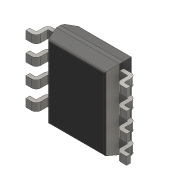
# Autodesk Inventor part: TCS3200
Saved by Autodesk Inventor 2016 (Build 200138000, 138)
## iProperties
Created: 2016-08-30
Part Number: TCS3200
Material: ABS Plastic
Document SubType Name: Modeling
Designer: Ádi
Density: 1.06 g/cm^3
Appearance: Semi-Polished
Mass: 0.0345678 g
Surface Area: 0.885583 cm^2
Volume: 0.0326111 cm^3
Author: Ádi
Autodesk Inventor part; units mm, degrees
ref_plane "YZ Plane" through (0, 0, 0) normal (1, 0, 0) x (0, 1, 0)
ref_plane "XZ Plane" through (0, 0, 0) normal (0, 1, 0) x (-1, 0, 0)
ref_plane "XY Plane" through (0, 0, 0) normal (0, 0, 1) x (1, 0, 0)
sketch "Sketch1" plane through (0, 0, 0) normal (0, 1, 0) x (-1, 0, 0)
  line L0 (-2, 2.5) -> (2, 2.5)
  line L1 (2, 2.5) -> (2, -2.5)
  line L2 (2, -2.5) -> (-2, -2.5)
  line L3 (-2, -2.5) -> (-2, 2.5)
  line L4 (-2, 2.5) -> (2, -2.5) construction
  line L5 (2, 2.5) -> (-2, -2.5) construction
  point P0 (0, 0)
  dimension "d0" = 4
  dimension "d1" = 5
  constraints: 12 end point, 2 midpoint, 2 parallel, 1 horizontal, 1 perpendicular
  measures "d0" distance of L1.end L2.end
  measures "d1" distance of L0.end L1.end
extrude "Extrusion1" add sketch "Sketch1" along normal blind 1.75
chamfer "Chamfer1" distance 0.5 angle 45 1 edges at (-2, 1.75, 0)
chamfer "Chamfer2" distance 0.2 angle 75 1 edges at (0, 0, 2.5) measured on face at (0.6667, 0, 0.8333)
chamfer "Chamfer3" distance 0.2 angle 75 1 edges at (2, 0, -0.1) measured on face at (0.6667, 0, 0.7)
chamfer "Chamfer4" distance 0.2 angle 75 1 edges at (-0.1, 0, -2.5) measured on face at (0.5333, 0, 0.7)
chamfer "Chamfer5" distance 0.2 angle 75 1 edges at (-2, 0, 0) measured on face at (0.5333, 0, 0.7667)
chamfer "Chamfer6" distance 0.2 angle 75 1 edges at (2, 1.75, 0) measured on face at (0.8333, 1.75, 0.8333)
chamfer "Chamfer7" distance 0.2 angle 75 1 edges at (0.15, 1.75, -2.5) measured on face at (0.7, 1.75, 0.8333)
chamfer "Chamfer8" distance 0.2 angle 75 1 edges at (0.15, 1.75, 2.5) measured on face at (0.7, 1.75, 0.9)
fillet "Fillet1" radius 0.1 7 edges at (0.15, 1.75, -2.3) (1.8, 1.75, 0) (0.15, 1.75, 2.3) (-1.8, 0, 0) (0, 0, 2.3) (1.8, 0, 0) (0, 0, -2.3)
sketch "Sketch2" plane through (0, 1.75, 0) normal (0, 1, 0) x (1, 0, 0)
  line L0 (-2, 2.434) -> (-2, -2.434) projected
  line L1 (2, 2.5) -> (-2, 2.5) projected
  line L2 (2, -2.5) -> (2, 2.5) projected
  line L3 (-2, -2.5) -> (2, -2.5) projected
  circle A0 centre (0, 0) radius 1.4
  dimension "d29" = 2.8
  constraints: 1 centre point, 1 coincident
  measures "d29" diameter of A0
extrude "Extrusion2" cut sketch "Sketch2" against normal blind 0.3
sketch "Sketch3" plane through (0, 1.45, 0) normal (0, 1, 0) x (1, 0, 0)
  circle A0 centre (0, 0) radius 1.4 projected
  line L0 (0.9822, -0.9977) -> (-0.9822, -0.9977)
  line L1 (-0.9822, -0.9977) -> (-0.9822, 0.9977)
  line L2 (-0.9822, 0.9977) -> (0.9822, 0.9977)
  line L3 (0.9822, 0.9977) -> (0.9822, -0.9977)
  line L4 (0.9822, -0.9977) -> (-0.9822, 0.9977) construction
  line L5 (-0.9822, -0.9977) -> (0.9822, 0.9977) construction
  constraints: 12 end point, 2 midpoint, 2 parallel, 1 horizontal, 1 perpendicular, 2 other
extrude "Extrusion3" add sketch "Sketch3" along normal blind 0.1 contours L3 L0 L1 L2
sketch "Sketch4" plane through (0, 1.55, 0) normal (0, 1, 0) x (1, 0, 0)
  line L0 (0.572, -0.5734) -> (-0.572, -0.5734)
  line L1 (-0.572, -0.5734) -> (-0.572, 0.5734)
  line L2 (-0.572, 0.5734) -> (0.572, 0.5734)
  line L3 (0.572, 0.5734) -> (0.572, -0.5734)
  line L4 (0.572, -0.5734) -> (-0.572, 0.5734) construction
  line L5 (-0.572, -0.5734) -> (0.572, 0.5734) construction
  point P0 (0, 0)
  constraints: 12 end point, 2 midpoint, 2 parallel, 1 horizontal, 1 perpendicular
extrude "Extrusion4" add sketch "Sketch4" along normal blind 0.1
sketch "Sketch5" plane through (-2, 0.7464, 2.5) normal (0, 0, 1) x (1, 0, 0)
  line L0 (0, 0.2572) -> (4, 0.2572) projected
  line L1 (0, 0) -> (0, 0.2572) projected
  line L2 (4, 0) -> (0, 0) projected
  line L3 (4, 0) -> (4, 0.2572) projected
  line L4 (4, 0.2572) -> (0, 0.2572) projected
  line L5 (0, 0.2572) -> (-0.79, 0.2572)
  line L6 (-1.2, -0.4964) -> (-1.2, -0.7464)
  line L7 (-1.2, -0.7464) -> (-0.54, -0.7464)
  line L8 (0, -0.7464) -> (0, 0.2572)
  line L9 (-1.2, -0.4964) -> (-0.79, -0.4964)
  line L10 (0, 0.0072) -> (-0.54, 0.0072)
  line L11 (-0.79, 0.2572) -> (-0.79, -0.4964)
  line L12 (-0.54, 0.0072) -> (-0.54, -0.7464)
  point P0 (2, -0.7464)
  dimension "d36" = 1.2
  dimension "d37" = 0.25
  dimension "d38" = 0.25
  dimension "d39" = 0.41
  dimension "d40" = 0.25
  constraints: 16 end point, 5 perpendicular, 2 parallel, 1 horizontal, 1 point on line
  measures "d36" distance of L8.start L6.end
  measures "d37" distance between parallel lines of L5 L10
  measures "d38" distance between parallel lines of L9 L7
  measures "d39" distance between parallel lines of L6 L11
  measures "d40" distance between parallel lines of L11 L12
extrude "Extrusion5" add sketch "Sketch5" against normal up to surface (5 mm away) contours L1 L10 L12 L7 L6 L9 L11 L5
fillet "Fillet2" radius 0.3 2 edges at (-2.79, 1.0036, 0) (-2.54, 0, 0)
fillet "Fillet3" radius 0.066 2 edges at (-2.79, 0.25, 0) (-2.54, 0.7536, 0)
sketch "Sketch6" plane through (-3.2, 0, -2.5) normal (0, -1, 0) x (1, 0, 0)
  line L0 (0.66, 5) -> (0.66, 0) projected
  line L1 (0, 5) -> (0, 0) projected
  line L2 (1.2, 5) -> (0.71, 5) projected
  line L3 (0, 4.62) -> (1.2, 4.62)
  line L4 (1.2, 4.62) -> (1.2, 5)
  line L5 (1.2, 5) -> (0, 5)
  line L6 (0, 5) -> (0, 4.62)
  line L7 (0, 3.375) -> (1.2, 3.375)
  line L8 (1.2, 3.375) -> (1.2, 4.12)
  line L9 (1.2, 4.12) -> (0, 4.12)
  line L10 (0, 4.12) -> (0, 3.375)
  line L11 (0, 2.875) -> (1.2, 2.875)
  line L12 (1.2, 2.875) -> (1.2, 2.13)
  line L13 (1.2, 2.13) -> (0, 2.13)
  line L14 (0, 2.13) -> (0, 2.875)
  line L15 (0, 1.63) -> (1.2, 1.63)
  line L16 (1.2, 1.63) -> (1.2, 0.885)
  line L17 (1.2, 0.885) -> (0, 0.885)
  line L18 (0, 0.885) -> (0, 1.63)
  line L19 (1.2, 5) -> (1.2, 0) projected
  line L20 (1.2, 0.385) -> (0, 0.385)
  line L21 (0, 0.385) -> (0, 0)
  line L22 (0, 0) -> (1.2, 0)
  line L23 (1.2, 0) -> (1.2, 0.385)
  line L24 (0, 0) -> (0.36, 0) projected
  point P0 (3.2, 2.5)
  dimension "d47" = 2.12
  dimension "d48" = 0.5
  dimension "d49" = 0.745
  dimension "d50" = 0.5
  dimension "d51" = 0.745
  dimension "d52" = 0.5
  dimension "d53" = 0.745
  dimension "d54" = 0.5
  dimension "d55" = 0
  constraints: 40 end point, 10 parallel, 6 point on line, 5 horizontal, 5 perpendicular
  measures "d47" distance from line of L3 point (3.2, 2.5)
  measures "d48" distance between parallel lines of L9 L3
  measures "d49" distance between parallel lines of L9 L7
  measures "d50" distance between parallel lines of L11 L7
  measures "d51" distance between parallel lines of L11 L13
  measures "d52" distance between parallel lines of L15 L13
  measures "d53" distance between parallel lines of L17 L15
  measures "d54" distance between parallel lines of L20 L17
  measures "d55" distance between parallel lines of L24 L22
extrude "Extrusion6" cut sketch "Sketch6" against normal through all contours L5 L2 L4 L3 L0 | L0 L3 L1 L5 | L9 L8 L7 L0 | L0 L7 L1 L9 | L11 L12 L13 L0 | L0 L13 L1 L11 | L15 L16 L17 L0 | L0 L17 L1 L15 | L20 L19 L22 L0 | L0 L22 L1 L20
mirror "Mirror1" about plane through (0, 0, 0) normal (1, 0, 0) of "Extrusion5", "Fillet3", "Extrusion6", "Fillet2"
body "Solid1"
